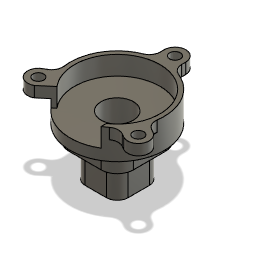
Miniscope_v4_Objective (Autodesk Fusion 360 design; units mm, degrees)
Autodesk Fusion 360 part; units mm, degrees
sketch "Sketch1" plane through (0, 0, 0) normal (0, 1, 0) x (1, 0, 0)
  circle A0 centre (0, 0) radius 1.5
  line L0 (-1, -2) -> (1, -2)
  line L1 (2, -1) -> (2, 1)
  line L2 (1, 2) -> (-1, 2)
  line L3 (-2, 1) -> (-2, -1)
  line L4 (-2, -2) -> (2, 2) construction
  line L5 (2, -2) -> (-2, 2) construction
  arc A1 (-1, 2) -> (-2, 1) centre (-1, 1) ccw
  arc A2 (-2, -1) -> (-1, -2) centre (-1, -1) ccw
  arc A3 (1, -2) -> (2, -1) centre (1, -1) ccw
  arc A4 (2, 1) -> (1, 2) centre (1, 1) ccw
  dimension "d1" = 3
  dimension "d2" = 1
  dimension "d3" = 1
  dimension "d50" = 2
  dimension "d51" = 2
  dimension "d52" = 4
  dimension "d53" = 4
  constraint coincident A0.centre origin
  constraint perpendicular L0 L1
  constraint parallel L0 L2
  constraint parallel L1 L3
  constraint horizontal L0
  constraint coincident L4 A0.centre
  constraint coincident L5 A0.centre
  constraint tangent L2 A1
  constraint tangent L3 A1
  constraint tangent L3 A2
  constraint tangent L0 A2
  constraint equal A1 A2
  constraint tangent L0 A3
  constraint tangent L1 A3
  constraint equal A1 A3
  constraint tangent L1 A4
  constraint tangent L2 A4
  measures "d1" diameter of A0
  measures "d2" radius of A1
  measures "d3" radius of A4
  measures "d50" distance of L3 A0.centre
  measures "d51" distance of A0.centre L2
  measures "d52" distance of L1 L3
  measures "d53" distance of L0 L2
extrude "Extrude1" add sketch "Sketch1" along normal blind 3
sketch "Sketch2" plane through (0, 3, 0) normal (0, 1, 0) x (-1, 0, 0)
  circle A0 centre (0, 0) radius 1.5
  arc A1 (-2, -1) -> (-1, -2) centre (-1, -1) ccw
  line L0 (-1, -2) -> (1, -2)
  arc A2 (1, -2) -> (2, -1) centre (1, -1) ccw
  line L1 (2, -1) -> (2, 1)
  arc A3 (2, 1) -> (1, 2) centre (1, 1) ccw
  line L2 (1, 2) -> (-1, 2)
  arc A4 (-1, 2) -> (-2, 1) centre (-1, 1) ccw
  line L3 (-2, 1) -> (-2, -1)
  line L4 (1.5, 3) -> (-1.5, 3)
  line L5 (-3, 1.5) -> (-3, -1.5)
  line L6 (-1.5, -3) -> (1.5, -3)
  line L7 (3, -1.5) -> (3, 1.5)
  line L8 (3, 3) -> (-3, -3) construction
  line L9 (-3, 3) -> (3, -3) construction
  arc A5 (1.5, -3) -> (3, -1.5) centre (1.5, -1.5) ccw
  arc A6 (3, 1.5) -> (1.5, 3) centre (1.5, 1.5) ccw
  arc A7 (-1.5, 3) -> (-3, 1.5) centre (-1.5, 1.5) ccw
  arc A8 (-3, -1.5) -> (-1.5, -3) centre (-1.5, -1.5) ccw
  dimension "d6" = 1.5
  constraint perpendicular L4 L5
  constraint parallel L4 L6
  constraint parallel L5 L7
  constraint horizontal L4
  constraint coincident L8 A0.centre
  constraint coincident L9 A0.centre
  constraint coincident A0.centre origin
  constraint tangent L6 A5
  constraint tangent L7 A5
  constraint tangent L7 A6
  constraint tangent L4 A6
  constraint equal A5 A6
  constraint tangent L4 A7
  constraint tangent L5 A7
  constraint equal A5 A7
  constraint tangent L5 A8
  constraint tangent L6 A8
  constraint equal A5 A8
  measures "d6" radius of A5
extrude "Extrude2" add sketch "Sketch2" along normal blind 1.5 contours A1 L0 A2 L1 A3 L2 A4 L3 | L4 L5 L6 L7 A5 A6 A7 A8
sketch "Sketch3" plane through (0, 4.5, 0) normal (0, 1, 0) x (-1, 0, 0)
  circle A0 centre (0, 0) radius 1.5
  arc A1 (-3, -1.5) -> (-1.5, -3) centre (-1.5, -1.5) ccw
  line L0 (-1.5, -3) -> (1.5, -3)
  arc A2 (1.5, -3) -> (3, -1.5) centre (1.5, -1.5) ccw
  line L1 (3, -1.5) -> (3, 1.5)
  arc A3 (3, 1.5) -> (1.5, 3) centre (1.5, 1.5) ccw
  line L2 (1.5, 3) -> (-1.5, 3)
  arc A4 (-1.5, 3) -> (-3, 1.5) centre (-1.5, 1.5) ccw
  line L3 (-3, 1.5) -> (-3, -1.5)
  line L4 (-1, -4.2592) -> (-1, -5.375)
  line L5 (0, -6.375) -> (0, -6.375)
  line L6 (1, -5.375) -> (1, -4.2592)
  circle A5 centre (0, -5.375) radius 0.5
  line L7 (0, 0) -> (0, -4.375) construction
  line L8 (0, -4.375) -> (0, -5.375) construction
  arc A6 (0, -6.375) -> (1, -5.375) centre (0, -5.375) ccw
  arc A7 (-1, -5.375) -> (0, -6.375) centre (0, -5.375) ccw
  arc A8 (5.1549, 1.8215) -> (5.5209, 3.1875) centre (4.6549, 2.6875) ccw
  line L9 (3.7889, 2.1875) -> (4.6549, 2.6875) construction
  circle A9 centre (4.6549, 2.6875) radius 0.5
  line L10 (4.1549, 3.5535) -> (3.1886, 2.9956)
  arc A10 (5.5209, 3.1875) -> (4.1549, 3.5535) centre (4.6549, 2.6875) ccw
  line L11 (5.5209, 3.1875) -> (5.5209, 3.1875)
  line L12 (4.1886, 1.2636) -> (5.1549, 1.8215)
  line L13 (0, 0) -> (3.7889, 2.1875) construction
  arc A11 (-4.1549, 3.5535) -> (-5.5209, 3.1875) centre (-4.6549, 2.6875) ccw
  line L14 (-3.7889, 2.1875) -> (-4.6549, 2.6875) construction
  circle A12 centre (-4.6549, 2.6875) radius 0.5
  line L15 (-5.1549, 1.8215) -> (-4.1886, 1.2636)
  arc A13 (-5.5209, 3.1875) -> (-5.1549, 1.8215) centre (-4.6549, 2.6875) ccw
  line L16 (-5.5209, 3.1875) -> (-5.5209, 3.1875)
  line L17 (-3.1886, 2.9956) -> (-4.1549, 3.5535)
  line L18 (0, 0) -> (-3.7889, 2.1875) construction
  arc A14 (1, -4.2592) -> (4.1886, 1.2636) centre (0, 0) ccw
  arc A15 (3.1886, 2.9956) -> (-3.1886, 2.9956) centre (0, 0) ccw
  arc A16 (-4.1886, 1.2636) -> (-1, -4.2592) centre (0, 0) ccw
  point P0 (-1, -6.375)
  point P1 (1, -6.375)
  point P2 (5.0209, 4.0535)
  point P3 (6.0209, 2.3215)
  point P4 (-6.0209, 2.3215)
  point P5 (-5.0209, 4.0535)
  dimension "d9" = 8.75
  dimension "d12" = 1
  dimension "d14" = 1
  dimension "d15" = 2
  dimension "d16" = 1
  dimension "d17" = 1
  dimension "d19" = 360
  constraint concentric A0 A14
  constraint vertical L4
  constraint vertical L6
  constraint coincident A0.centre L7.start
  constraint coincident A5.centre L8.end
  constraint parallel L7 L8
  constraint coincident P1 L6
  constraint tangent L6 A6
  constraint coincident P0 L5
  constraint coincident P0 L4
  constraint tangent L4 A7
  constraint concentric A14 A15
  constraint concentric A15 A16
  measures "d9" diameter of A14
  measures "d12" diameter of A5
  measures "d14" distance of A5.centre L7.end
  measures "d15" distance of P0 P1
  measures "d16" radius of A6
  measures "d17" radius of A7
extrude "Extrude3" add sketch "Sketch3" along normal blind 1 contours A1 L0 A2 L1 A3 L2 A4 L3 | L4 L6 A6 A7 A8 L10 A10 L12 A11 L15 A13 L17 A14 A15 A16
fillet "Fillet1" radius 1 6 edges at (3.1886, 5, 2.9956) (-3.1886, 5, 2.9956) (-4.1886, 5, 1.2636) (-1, 5, -4.2592) (1, 5, -4.2592) (4.1886, 5, 1.2636)
sketch "Sketch4" plane through (0, 5.5, 0) normal (0, 1, 0) x (-1, 0, 0)
  circle A0 centre (-4.6549, 2.6875) radius 0.5
  circle A1 centre (0, -5.375) radius 0.5
  circle A2 centre (0, 0) radius 1.5
  circle A3 centre (4.6549, 2.6875) radius 0.5
  arc A4 (-4.3308, 0.6206) -> (-1.6279, -4.0609) centre (0, 0) ccw
  arc A5 (-1, -4.9891) -> (-1.6279, -4.0609) centre (-2, -4.9891) ccw
  line L0 (-1, -4.9891) -> (-1, -5.375)
  arc A6 (-1, -5.375) -> (1, -5.375) centre (0, -5.375) ccw
  line L1 (1, -5.375) -> (1, -4.9891)
  arc A7 (1.6279, -4.0609) -> (1, -4.9891) centre (2, -4.9891) ccw
  arc A8 (1.6279, -4.0609) -> (4.3308, 0.6206) centre (0, 0) ccw
  arc A9 (4.8206, 1.6285) -> (4.3308, 0.6206) centre (5.3206, 0.7625) ccw
  line L2 (4.8206, 1.6285) -> (5.1549, 1.8215)
  arc A10 (5.1549, 1.8215) -> (4.1549, 3.5535) centre (4.6549, 2.6875) ccw
  line L3 (4.1549, 3.5535) -> (3.8206, 3.3606)
  arc A11 (2.7029, 3.4402) -> (3.8206, 3.3606) centre (3.3206, 4.2266) ccw
  arc A12 (2.7029, 3.4402) -> (-2.7029, 3.4402) centre (0, 0) ccw
  arc A13 (-3.8206, 3.3606) -> (-2.7029, 3.4402) centre (-3.3206, 4.2266) ccw
  line L4 (-3.8206, 3.3606) -> (-4.1549, 3.5535)
  arc A14 (-4.1549, 3.5535) -> (-5.1549, 1.8215) centre (-4.6549, 2.6875) ccw
  line L5 (-5.1549, 1.8215) -> (-4.8206, 1.6285)
  arc A15 (-4.3308, 0.6206) -> (-4.8206, 1.6285) centre (-5.3206, 0.7625) ccw
  circle A16 centre (0, 0) radius 3.975
  dimension "d23" = 7.95
  constraint concentric A2 A16
  measures "d23" diameter of A16
extrude "Extrude4" add sketch "Sketch4" along normal blind 1.75 contours A4 A5 L0 A6 L1 A7 A8 A9 L2 A10 L3 A11 A12 A13 L4 A14 L5 A15
sketch "Sketch5" plane through (0, 7.25, 0) normal (0, 1, 0) x (-1, 0, 0)
  circle A0 centre (4.6549, 2.6875) radius 0.5
  circle A1 centre (0, -5.375) radius 0.5
  circle A2 centre (-4.6549, 2.6875) radius 0.5
  circle A3 centre (0, 0) radius 3.975
  line L0 (-1, -4.9891) -> (-1, -5.375)
  arc A4 (-1, -5.375) -> (1, -5.375) centre (0, -5.375) ccw
  line L1 (1, -5.375) -> (1, -4.9891)
  arc A5 (1.6279, -4.0609) -> (1, -4.9891) centre (2, -4.9891) ccw
  arc A6 (1.6279, -4.0609) -> (4.3308, 0.6206) centre (0, 0) ccw
  arc A7 (4.8206, 1.6285) -> (4.3308, 0.6206) centre (5.3206, 0.7625) ccw
  line L2 (4.8206, 1.6285) -> (5.1549, 1.8215)
  arc A8 (5.1549, 1.8215) -> (4.1549, 3.5535) centre (4.6549, 2.6875) ccw
  line L3 (4.1549, 3.5535) -> (3.8206, 3.3606)
  arc A9 (2.7029, 3.4402) -> (3.8206, 3.3606) centre (3.3206, 4.2266) ccw
  arc A10 (2.7029, 3.4402) -> (-2.7029, 3.4402) centre (0, 0) ccw
  arc A11 (-3.8206, 3.3606) -> (-2.7029, 3.4402) centre (-3.3206, 4.2266) ccw
  line L4 (-3.8206, 3.3606) -> (-4.1549, 3.5535)
  arc A12 (-4.1549, 3.5535) -> (-5.1549, 1.8215) centre (-4.6549, 2.6875) ccw
  line L5 (-5.1549, 1.8215) -> (-4.8206, 1.6285)
  arc A13 (-4.3308, 0.6206) -> (-4.8206, 1.6285) centre (-5.3206, 0.7625) ccw
  arc A14 (-4.3308, 0.6206) -> (-1.6279, -4.0609) centre (0, 0) ccw
  arc A15 (-1, -4.9891) -> (-1.6279, -4.0609) centre (-2, -4.9891) ccw
  line L6 (2.25, 4.375) -> (-2.25, 4.375)
  line L7 (-2.25, 4.375) -> (-2.25, 3.2769)
  line L8 (-2.25, 3.2769) -> (2.25, 3.2769) construction
  line L9 (2.25, 3.2769) -> (2.25, 4.375) construction
  line L10 (2.25, 4.375) -> (-2.25, 3.2769) construction
  line L11 (-2.25, 4.375) -> (2.25, 3.2769) construction
  line L12 (0, 0) -> (-2.25, 3.2769)
  line L13 (0, 0) -> (4.1549, 3.5535)
  line L14 (2.25, 4.375) -> (4.1549, 3.5535)
  point P0 (0, 3.826)
  dimension "d49" = 2.25
  constraint perpendicular L6 L7
  constraint parallel L6 L8
  constraint parallel L7 L9
  constraint horizontal L6
  constraint coincident L10 P0
  constraint coincident L11 P0
  constraint midpoint L11 P0
  constraint coincident A3 L8.end
  constraint tangent A10 L6
  constraint coincident A3 L7.end
  constraint coincident A3.centre A6.centre
  constraint coincident A8.end L3.start
  measures "d49" distance of A3.centre L7
extrude "Extrude5" cut sketch "Sketch5" against normal up to surface (1.75 mm away) contours A3 L12 L13 | A3 L3 A9 A10 L7 L13 | A3 L12 L13
sketch "Sketch8" plane through (0, 4.5, 0) normal (0, -1, 0) x (1, 0, 0)
  arc A0 (4.8206, 1.6285) -> (4.3308, 0.6206) centre (5.3206, 0.7625) ccw
  line L0 (4.8206, 1.6285) -> (5.1549, 1.8215)
  arc A1 (5.1549, 1.8215) -> (4.1549, 3.5535) centre (4.6549, 2.6875) ccw
  line L1 (4.1549, 3.5535) -> (3.8206, 3.3606)
  arc A2 (2.7029, 3.4402) -> (3.8206, 3.3606) centre (3.3206, 4.2266) ccw
  arc A3 (2.7029, 3.4402) -> (-2.7029, 3.4402) centre (0, 0) ccw
  arc A4 (-3.8206, 3.3606) -> (-2.7029, 3.4402) centre (-3.3206, 4.2266) ccw
  line L2 (-3.8206, 3.3606) -> (-4.1549, 3.5535)
  arc A5 (-4.1549, 3.5535) -> (-5.1549, 1.8215) centre (-4.6549, 2.6875) ccw
  line L3 (-5.1549, 1.8215) -> (-4.8206, 1.6285)
  arc A6 (-4.3308, 0.6206) -> (-4.8206, 1.6285) centre (-5.3206, 0.7625) ccw
  arc A7 (-4.3308, 0.6206) -> (-1.6279, -4.0609) centre (0, 0) ccw
  arc A8 (-1, -4.9891) -> (-1.6279, -4.0609) centre (-2, -4.9891) ccw
  line L4 (-1, -4.9891) -> (-1, -5.375)
  arc A9 (-1, -5.375) -> (1, -5.375) centre (0, -5.375) ccw
  line L5 (1, -5.375) -> (1, -4.9891)
  arc A10 (1.6279, -4.0609) -> (1, -4.9891) centre (2, -4.9891) ccw
  arc A11 (1.6279, -4.0609) -> (4.3308, 0.6206) centre (0, 0) ccw
  circle A12 centre (-4.6549, 2.6875) radius 0.5
  circle A13 centre (0, -5.375) radius 0.5
  circle A14 centre (4.6549, 2.6875) radius 0.5
  line L6 (3, 1.5) -> (3, -1.5)
  arc A15 (1.5, -3) -> (3, -1.5) centre (1.5, -1.5) ccw
  line L7 (1.5, -3) -> (-1.5, -3)
  arc A16 (-3, -1.5) -> (-1.5, -3) centre (-1.5, -1.5) ccw
  line L8 (-3, -1.5) -> (-3, 1.5)
  arc A17 (-1.5, 3) -> (-3, 1.5) centre (-1.5, 1.5) ccw
  line L9 (-1.5, 3) -> (1.5, 3)
  arc A18 (3, 1.5) -> (1.5, 3) centre (1.5, 1.5) ccw
  circle A19 centre (0, 0) radius 4.375
  constraint coincident A3.centre A7.centre
  constraint coincident A6.start A19
extrude "Extrude6" cut sketch "Sketch8" against normal up to surface (1.75 mm away) contours A0 L0 A1 L1 A2 A19 | A8 L4 A9 L5 A10 A19 | A4 L2 A5 L3 A6 A19
